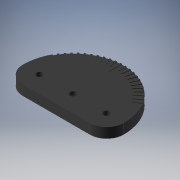
# Autodesk Inventor part: Angled Sensor Mount Base
Saved by Autodesk Inventor 2019 (Build 230136000, 136)
## iProperties
Created: 2019-01-21
Part Number: Angled Sensor Mount Base
Material: Generic
Document SubType Name: Modeling
Designer: Billy
Density: 1 g/cm^3
Appearance: Default
Author: Billy
Autodesk Inventor part; units mm, degrees
ref_plane "YZ Plane" through (0, 0, 0) normal (1, 0, 0) x (0, 1, 0)
ref_plane "XZ Plane" through (0, 0, 0) normal (0, 1, 0) x (-1, 0, 0)
ref_plane "XY Plane" through (0, 0, 0) normal (0, 0, 1) x (1, 0, 0)
sketch "Sketch1" plane through (0, 0, 0) normal (0, 1, 0) x (-1, 0, 0)
  circle A0 centre (0, 0) radius 2
  arc A1 (0, 10) -> (0, -10) centre (0, 0) ccw
  circle A2 centre (40, 0) radius 2
  arc A3 (40, -10) -> (40, 10) centre (40, 0) ccw
  line L0 (40, 10) -> (0, 10)
  line L1 (40, -10) -> (0, -10)
  circle A4 centre (20, 0) radius 2
  dimension "d0" = 4
  dimension "d1" = 20
  dimension "d2" = 4
  dimension "d3" = 20
  dimension "d4" = 4
  constraints: 5 centre point, 4 end point, 4 point on circle, 3 coincident, 1 parallel, 1 tangent
  measures "d0" diameter of A0
  measures "d1" diameter of A1
  measures "d2" diameter of A2
  measures "d3" diameter of A3
  measures "d4" diameter of A4
extrude "Extrusion1" add sketch "Sketch1" along normal blind 6
sketch "Sketch2" plane through (0, 0, 0) normal (0, -1, 0) x (1, 0, 0)
  circle A0 centre (-20, 0) radius 2 projected
  circle A1 centre (-40, 0) radius 2 projected
  circle A2 centre (0, 0) radius 2 projected
  arc A3 (-40, 10) -> (-40, -10) centre (-40, 0) ccw projected
  line L0 (-40, -10) -> (0, -10) projected
  arc A4 (0, -10) -> (0, 10) centre (0, 0) ccw projected
  line L1 (0, 10) -> (-40, 10) projected
  circle A5 centre (-20, 0) radius 5
  dimension "d7" = 10
  constraints: 1 centre point, 1 coincident
  measures "d7" diameter of A5
extrude "Extrusion2" cut sketch "Sketch2" against normal blind 4 contours A5
sketch "Sketch3" plane through (0, 6, 0) normal (0, 1, 0) x (1, 0, 0)
  circle A0 centre (-20, 0) radius 2
  circle A1 centre (-40, 0) radius 2
  circle A2 centre (0, 0) radius 2
  arc A3 (-40, 10) -> (-50, 0) centre (-40, 0) ccw
  line L0 (-40, -10) -> (0, -10)
  arc A4 (10, 0) -> (0, 10) centre (0, 0) ccw
  line L1 (0, 10) -> (-40, 10)
  arc A5 (10, 0) -> (-50, 0) centre (-20, 0) ccw
  constraints: 10 centre point, 6 point on circle, 4 end point, 1 coincident
extrude "Extrusion3" add sketch "Sketch3" against normal up to surface (6 mm away) contours A3 A5 A4 L1
sketch "Sketch4" plane through (0, 6, 0) normal (0, 1, 0) x (1, 0, 0)
  circle A0 centre (-20, 0) radius 2
  circle A1 centre (-40, 0) radius 2
  circle A2 centre (0, 0) radius 2
  arc A3 (-50, 0) -> (-40, -10) centre (-40, 0) ccw
  line L0 (-40, -10) -> (0, -10)
  arc A4 (0, -10) -> (10, 0) centre (0, 0) ccw
  arc A5 (-19, 29.9833) -> (-20, 30) centre (-20, 0) ccw
  arc A6 (-19, 29.9833) -> (-21, 29.9833) centre (-20, 0) ccw
  line L1 (-21, 29.9833) -> (-21, 25)
  line L2 (-21, 25) -> (-20, 25)
  line L3 (-19, 29.9833) -> (-19, 25)
  line L4 (-19, 25) -> (-20, 25)
  arc A7 (-21.8546, 29.9426) -> (-22.8517, 29.8642) centre (-20, 0) ccw
  arc A8 (-21.8546, 29.9426) -> (-23.8456, 29.7525) centre (-20, 0) ccw
  line L5 (-23.8456, 29.7525) -> (-23.3719, 24.7917)
  line L6 (-23.3719, 24.7917) -> (-22.3764, 24.8868)
  line L7 (-21.8546, 29.9426) -> (-21.3809, 24.9819)
  line L8 (-21.3809, 24.9819) -> (-22.3764, 24.8868)
  arc A9 (-24.6925, 29.6307) -> (-25.6775, 29.4579) centre (-20, 0) ccw
  arc A10 (-24.6925, 29.6307) -> (-26.6563, 29.2522) centre (-20, 0) ccw
  line L9 (-26.6563, 29.2522) -> (-25.7132, 24.359)
  line L10 (-25.7132, 24.359) -> (-24.7313, 24.5482)
  line L11 (-24.6925, 29.6307) -> (-23.7494, 24.7375)
  line L12 (-23.7494, 24.7375) -> (-24.7313, 24.5482)
  arc A11 (-27.4878, 29.0505) -> (-28.452, 28.7848) centre (-20, 0) ccw
  arc A12 (-27.4878, 29.0505) -> (-29.4068, 28.4871) centre (-20, 0) ccw
  line L13 (-29.4068, 28.4871) -> (-28.0028, 23.7056)
  line L14 (-28.0028, 23.7056) -> (-27.0433, 23.9873)
  line L15 (-27.4878, 29.0505) -> (-26.0838, 24.2691)
  line L16 (-26.0838, 24.2691) -> (-27.0433, 23.9873)
  arc A13 (-30.2153, 28.2072) -> (-31.1499, 27.851) centre (-20, 0) ccw
  arc A14 (-30.2153, 28.2072) -> (-32.072, 27.4639) centre (-20, 0) ccw
  line L17 (-32.072, 27.4639) -> (-30.2199, 22.8375)
  line L18 (-30.2199, 22.8375) -> (-29.2916, 23.2092)
  line L19 (-30.2153, 28.2072) -> (-28.3632, 23.5809)
  line L20 (-28.3632, 23.5809) -> (-29.2916, 23.2092)
  arc A15 (-32.8503, 27.1085) -> (-33.7468, 26.6651) centre (-20, 0) ccw
  arc A16 (-32.8503, 27.1085) -> (-34.628, 26.192) centre (-20, 0) ccw
  line L21 (-34.628, 26.192) -> (-32.3445, 21.7627)
  line L22 (-32.3445, 21.7627) -> (-31.4557, 22.2209)
  line L23 (-32.8503, 27.1085) -> (-30.5668, 22.6791)
  line L24 (-30.5668, 22.6791) -> (-31.4557, 22.2209)
  arc A17 (-35.369, 25.7642) -> (-36.2192, 25.2376) centre (-20, 0) ccw
  arc A18 (-35.369, 25.7642) -> (-37.0515, 24.6829) centre (-20, 0) ccw
  line L25 (-37.0515, 24.6829) -> (-34.3573, 20.4907)
  line L26 (-34.3573, 20.4907) -> (-33.516, 21.0313)
  line L27 (-35.369, 25.7642) -> (-32.6748, 21.572)
  line L28 (-32.6748, 21.572) -> (-33.516, 21.0313)
  arc A19 (-37.7484, 24.1866) -> (-38.5448, 23.5816) centre (-20, 0) ccw
  arc A20 (-37.7484, 24.1866) -> (-39.3205, 22.9503) centre (-20, 0) ccw
  line L29 (-39.3205, 22.9503) -> (-36.24, 19.0332)
  line L30 (-36.24, 19.0332) -> (-35.454, 19.6513)
  line L31 (-37.7484, 24.1866) -> (-34.6679, 20.2695)
  line L32 (-34.6679, 20.2695) -> (-35.454, 19.6513)
  arc A21 (-39.9671, 22.39) -> (-40.7024, 21.712) centre (-20, 0) ccw
  arc A22 (-39.9671, 22.39) -> (-41.4146, 21.0099) centre (-20, 0) ccw
  line L33 (-41.4146, 21.0099) -> (-37.9757, 17.4033)
  line L34 (-37.9757, 17.4033) -> (-37.252, 18.0934)
  line L35 (-39.9671, 22.39) -> (-36.5282, 18.7834)
  line L36 (-36.5282, 18.7834) -> (-37.252, 18.0934)
  arc A23 (-42.005, 20.3907) -> (-42.6725, 19.6458) centre (-20, 0) ccw
  arc A24 (-42.005, 20.3907) -> (-43.3147, 18.8792) centre (-20, 0) ccw
  line L37 (-43.3147, 18.8792) -> (-39.5486, 15.6158)
  line L38 (-39.5486, 15.6158) -> (-38.8937, 16.3715)
  line L39 (-42.005, 20.3907) -> (-38.2389, 17.1273)
  line L40 (-38.2389, 17.1273) -> (-38.8937, 16.3715)
  arc A25 (-43.8436, 18.2066) -> (-44.4373, 17.4017) centre (-20, 0) ccw
  arc A26 (-43.8436, 18.2066) -> (-45.0038, 16.5775) centre (-20, 0) ccw
  line L41 (-45.0038, 16.5775) -> (-40.9445, 13.6868)
  line L42 (-40.9445, 13.6868) -> (-40.3644, 14.5014)
  line L43 (-43.8436, 18.2066) -> (-39.7843, 15.316)
  line L44 (-39.7843, 15.316) -> (-40.3644, 14.5014)
  arc A27 (-45.4663, 15.8577) -> (-45.9808, 15) centre (-20, 0) ccw
  arc A28 (-45.4663, 15.8577) -> (-46.4663, 14.1256) centre (-20, 0) ccw
  line L45 (-46.4663, 14.1256) -> (-42.1506, 11.634)
  line L46 (-42.1506, 11.634) -> (-41.6506, 12.5)
  line L47 (-45.4663, 15.8577) -> (-41.1506, 13.366)
  line L48 (-41.1506, 13.366) -> (-41.6506, 12.5)
  arc A29 (-16.1544, 29.7525) -> (-17.1483, 29.8642) centre (-20, 0) ccw
  arc A30 (-16.1544, 29.7525) -> (-18.1454, 29.9426) centre (-20, 0) ccw
  line L49 (-18.1454, 29.9426) -> (-18.6191, 24.9819)
  line L50 (-18.6191, 24.9819) -> (-17.6236, 24.8868)
  line L51 (-16.6281, 24.7917) -> (-17.6236, 24.8868)
  line L52 (-16.1544, 29.7525) -> (-16.6281, 24.7917)
  arc A31 (-13.3437, 29.2522) -> (-14.3225, 29.4579) centre (-20, 0) ccw
  arc A32 (-13.3437, 29.2522) -> (-15.3075, 29.6307) centre (-20, 0) ccw
  line L53 (-15.3075, 29.6307) -> (-16.2506, 24.7375)
  line L54 (-16.2506, 24.7375) -> (-15.2687, 24.5482)
  line L55 (-14.2868, 24.359) -> (-15.2687, 24.5482)
  line L56 (-13.3437, 29.2522) -> (-14.2868, 24.359)
  arc A33 (-10.5932, 28.4871) -> (-11.548, 28.7848) centre (-20, 0) ccw
  arc A34 (-10.5932, 28.4871) -> (-12.5122, 29.0505) centre (-20, 0) ccw
  line L57 (-12.5122, 29.0505) -> (-13.9162, 24.2691)
  line L58 (-13.9162, 24.2691) -> (-12.9567, 23.9873)
  line L59 (-11.9972, 23.7056) -> (-12.9567, 23.9873)
  line L60 (-10.5932, 28.4871) -> (-11.9972, 23.7056)
  arc A35 (-7.928, 27.4639) -> (-8.8501, 27.851) centre (-20, 0) ccw
  arc A36 (-7.928, 27.4639) -> (-9.7847, 28.2072) centre (-20, 0) ccw
  line L61 (-9.7847, 28.2072) -> (-11.6368, 23.5809)
  line L62 (-11.6368, 23.5809) -> (-10.7084, 23.2092)
  line L63 (-9.7801, 22.8375) -> (-10.7084, 23.2092)
  line L64 (-7.928, 27.4639) -> (-9.7801, 22.8375)
  arc A37 (-5.372, 26.192) -> (-6.2532, 26.6651) centre (-20, 0) ccw
  arc A38 (-5.372, 26.192) -> (-7.1497, 27.1085) centre (-20, 0) ccw
  line L65 (-7.1497, 27.1085) -> (-9.4332, 22.6791)
  line L66 (-9.4332, 22.6791) -> (-8.5443, 22.2209)
  line L67 (-7.6555, 21.7627) -> (-8.5443, 22.2209)
  line L68 (-5.372, 26.192) -> (-7.6555, 21.7627)
  arc A39 (-2.9485, 24.6829) -> (-3.7808, 25.2376) centre (-20, 0) ccw
  arc A40 (-2.9485, 24.6829) -> (-4.631, 25.7642) centre (-20, 0) ccw
  line L69 (-4.631, 25.7642) -> (-7.3252, 21.572)
  line L70 (-7.3252, 21.572) -> (-6.484, 21.0313)
  line L71 (-5.6427, 20.4907) -> (-6.484, 21.0313)
  line L72 (-2.9485, 24.6829) -> (-5.6427, 20.4907)
  arc A41 (-0.6795, 22.9503) -> (-1.4552, 23.5816) centre (-20, 0) ccw
  arc A42 (-0.6795, 22.9503) -> (-2.2516, 24.1866) centre (-20, 0) ccw
  line L73 (-2.2516, 24.1866) -> (-5.3321, 20.2695)
  line L74 (-5.3321, 20.2695) -> (-4.546, 19.6513)
  line L75 (-3.76, 19.0332) -> (-4.546, 19.6513)
  line L76 (-0.6795, 22.9503) -> (-3.76, 19.0332)
  arc A43 (1.4146, 21.0099) -> (0.7024, 21.712) centre (-20, 0) ccw
  arc A44 (1.4146, 21.0099) -> (-0.0329, 22.39) centre (-20, 0) ccw
  line L77 (-0.0329, 22.39) -> (-3.4718, 18.7834)
  line L78 (-3.4718, 18.7834) -> (-2.748, 18.0934)
  line L79 (-2.0243, 17.4033) -> (-2.748, 18.0934)
  line L80 (1.4146, 21.0099) -> (-2.0243, 17.4033)
  arc A45 (3.3147, 18.8792) -> (2.6725, 19.6458) centre (-20, 0) ccw
  arc A46 (3.3147, 18.8792) -> (2.005, 20.3907) centre (-20, 0) ccw
  line L81 (2.005, 20.3907) -> (-1.7611, 17.1273)
  line L82 (-1.7611, 17.1273) -> (-1.1063, 16.3715)
  line L83 (-0.4514, 15.6158) -> (-1.1063, 16.3715)
  line L84 (3.3147, 18.8792) -> (-0.4514, 15.6158)
  arc A47 (5.0038, 16.5775) -> (4.4373, 17.4017) centre (-20, 0) ccw
  arc A48 (5.0038, 16.5775) -> (3.8436, 18.2066) centre (-20, 0) ccw
  line L85 (3.8436, 18.2066) -> (-0.2157, 15.316)
  line L86 (-0.2157, 15.316) -> (0.3644, 14.5014)
  line L87 (0.9445, 13.6868) -> (0.3644, 14.5014)
  line L88 (5.0038, 16.5775) -> (0.9445, 13.6868)
  arc A49 (6.4663, 14.1256) -> (5.9808, 15) centre (-20, 0) ccw
  arc A50 (6.4663, 14.1256) -> (5.4663, 15.8577) centre (-20, 0) ccw
  line L89 (5.4663, 15.8577) -> (1.1506, 13.366)
  line L90 (1.1506, 13.366) -> (1.6506, 12.5)
  line L91 (2.1506, 11.634) -> (1.6506, 12.5)
  line L92 (6.4663, 14.1256) -> (2.1506, 11.634)
  point P0 (-19, 25)
  point P1 (-16.6281, 24.7917)
  point P2 (-9.7801, 22.8375)
  point P3 (-7.6555, 21.7627)
  point P4 (-5.6427, 20.4907)
  point P5 (-3.76, 19.0332)
  point P6 (-2.0243, 17.4033)
  point P7 (0.9445, 13.6868)
  dimension "d17" = 60
  dimension "d21" = 60
  constraints: 186 end point, 119 point on circle, 78 centre point, 321 other
extrude "Extrusion4" cut sketch "Sketch4" against normal blind 0.5 contours L3 L4 L2 L1 A6 A5 | L7 L8 L6 L5 A8 A7 | L11 L12 L10 L9 A10 A9 | L15 L16 L14 L13 A12 A11 | L19 L20 L18 L17 A14 A13 | L23 L24 L22 L21 A16 A15 | L27 L28 L26 L25 A18 A17 | L31 L32 L30 L29 A20 A19 | L35 L36 L34 L33 A22 A21 | L39 L40 L38 L37 A24 A23 | L43 L44 L42 L41 A26 A25 | L47 L48 L46 L45 A28 A27 | L52 L51 L50 L49 A30 A29 | L56 L55 L54 L53 A32 A31 | L60 L59 L58 L57 A34 A33 | L64 L63 L62 L61 A36 A35 | L68 L67 L66 L65 A38 A37 | L72 L71 L70 L69 A40 A39 | L76 L75 L74 L73 A42 A41 | L80 L79 L78 L77 A44 A43 | L84 L83 L82 L81 A46 A45 | L88 L87 L86 L85 A48 A47 | L92 L91 L90 L89 A50 A49
sketch "Sketch5" plane through (0, 6, 0) normal (0, 1, 0) x (1, 0, 0)
  line L0 (-16.2506, 24.7375) -> (-15.3075, 29.6307) projected
  arc A0 (-15.3075, 29.6307) -> (-16.1544, 29.7525) centre (-20, 0) ccw projected
  line L1 (-16.1544, 29.7525) -> (-16.6281, 24.7917) projected
  line L2 (-16.6281, 24.7917) -> (-18.6191, 24.9819) projected
  line L3 (-18.6191, 24.9819) -> (-18.1454, 29.9426) projected
  arc A1 (-18.1454, 29.9426) -> (-19, 29.9833) centre (-20, 0) ccw projected
  line L4 (-19, 29.9833) -> (-19, 25) projected
  line L5 (-19, 25) -> (-21, 25) projected
  line L6 (-21, 25) -> (-21, 29.9833) projected
  arc A2 (-21, 29.9833) -> (-21.8546, 29.9426) centre (-20, 0) ccw projected
  line L7 (-21.8546, 29.9426) -> (-21.3809, 24.9819) projected
  line L8 (-21.3809, 24.9819) -> (-23.3719, 24.7917) projected
  line L9 (-23.3719, 24.7917) -> (-23.8456, 29.7525) projected
  arc A3 (-23.8456, 29.7525) -> (-24.6925, 29.6307) centre (-20, 0) ccw projected
  line L10 (-24.6925, 29.6307) -> (-23.7494, 24.7375) projected
  line L11 (-23.7494, 24.7375) -> (-25.7132, 24.359) projected
  line L12 (-25.7132, 24.359) -> (-26.6563, 29.2522) projected
  arc A4 (-26.6563, 29.2522) -> (-27.4878, 29.0505) centre (-20, 0) ccw projected
  line L13 (-27.4878, 29.0505) -> (-26.0838, 24.2691) projected
  line L14 (-26.0838, 24.2691) -> (-28.0028, 23.7056) projected
  line L15 (-28.0028, 23.7056) -> (-29.4068, 28.4871) projected
  arc A5 (-29.4068, 28.4871) -> (-30.2153, 28.2072) centre (-20, 0) ccw projected
  line L16 (-30.2153, 28.2072) -> (-28.3632, 23.5809) projected
  line L17 (-28.3632, 23.5809) -> (-30.2199, 22.8375) projected
  line L18 (-30.2199, 22.8375) -> (-32.072, 27.4639) projected
  arc A6 (-32.072, 27.4639) -> (-32.8503, 27.1085) centre (-20, 0) ccw projected
  line L19 (-32.8503, 27.1085) -> (-30.5668, 22.6791) projected
  line L20 (-30.5668, 22.6791) -> (-32.3445, 21.7627) projected
  line L21 (-32.3445, 21.7627) -> (-34.628, 26.192) projected
  arc A7 (-34.628, 26.192) -> (-35.369, 25.7642) centre (-20, 0) ccw projected
  line L22 (-35.369, 25.7642) -> (-32.6748, 21.572) projected
  line L23 (-32.6748, 21.572) -> (-34.3573, 20.4907) projected
  line L24 (-34.3573, 20.4907) -> (-37.0515, 24.6829) projected
  arc A8 (-37.0515, 24.6829) -> (-37.7484, 24.1866) centre (-20, 0) ccw projected
  line L25 (-37.7484, 24.1866) -> (-34.6679, 20.2695) projected
  line L26 (-34.6679, 20.2695) -> (-36.24, 19.0332) projected
  line L27 (-36.24, 19.0332) -> (-39.3205, 22.9503) projected
  arc A9 (-39.3205, 22.9503) -> (-39.9671, 22.39) centre (-20, 0) ccw projected
  line L28 (-39.9671, 22.39) -> (-36.5282, 18.7834) projected
  line L29 (-36.5282, 18.7834) -> (-37.9757, 17.4033) projected
  line L30 (-37.9757, 17.4033) -> (-41.4146, 21.0099) projected
  arc A10 (-41.4146, 21.0099) -> (-42.005, 20.3907) centre (-20, 0) ccw projected
  line L31 (-42.005, 20.3907) -> (-38.2389, 17.1273) projected
  line L32 (-38.2389, 17.1273) -> (-39.5486, 15.6158) projected
  line L33 (-39.5486, 15.6158) -> (-43.3147, 18.8792) projected
  arc A11 (-43.3147, 18.8792) -> (-43.8436, 18.2066) centre (-20, 0) ccw projected
  line L34 (-43.8436, 18.2066) -> (-39.7843, 15.316) projected
  line L35 (-39.7843, 15.316) -> (-40.9445, 13.6868) projected
  line L36 (-40.9445, 13.6868) -> (-45.0038, 16.5775) projected
  arc A12 (-45.0038, 16.5775) -> (-45.4663, 15.8577) centre (-20, 0) ccw projected
  line L37 (-45.4663, 15.8577) -> (-41.1506, 13.366) projected
  line L38 (-41.1506, 13.366) -> (-42.1506, 11.634) projected
  line L39 (-42.1506, 11.634) -> (-46.4663, 14.1256) projected
  arc A13 (-46.4663, 14.1256) -> (-50, 0) centre (-20, 0) ccw projected
  arc A14 (-50, 0) -> (-40, -10) centre (-40, 0) ccw projected
  line L40 (-40, -10) -> (0, -10) projected
  arc A15 (0, -10) -> (10, 0) centre (0, 0) ccw projected
  arc A16 (10, 0) -> (6.4663, 14.1256) centre (-20, 0) ccw projected
  line L41 (6.4663, 14.1256) -> (2.1506, 11.634) projected
  line L42 (2.1506, 11.634) -> (1.1506, 13.366) projected
  line L43 (1.1506, 13.366) -> (5.4663, 15.8577) projected
  arc A17 (5.4663, 15.8577) -> (5.0038, 16.5775) centre (-20, 0) ccw projected
  line L44 (5.0038, 16.5775) -> (0.9445, 13.6868) projected
  line L45 (0.9445, 13.6868) -> (-0.2157, 15.316) projected
  line L46 (-0.2157, 15.316) -> (3.8436, 18.2066) projected
  arc A18 (3.8436, 18.2066) -> (3.3147, 18.8792) centre (-20, 0) ccw projected
  line L47 (3.3147, 18.8792) -> (-0.4514, 15.6158) projected
  line L48 (-0.4514, 15.6158) -> (-1.7611, 17.1273) projected
  line L49 (-1.7611, 17.1273) -> (2.005, 20.3907) projected
  arc A19 (2.005, 20.3907) -> (1.4146, 21.0099) centre (-20, 0) ccw projected
  line L50 (1.4146, 21.0099) -> (-2.0243, 17.4033) projected
  line L51 (-2.0243, 17.4033) -> (-3.4718, 18.7834) projected
  line L52 (-3.4718, 18.7834) -> (-0.0329, 22.39) projected
  arc A20 (-0.0329, 22.39) -> (-0.6795, 22.9503) centre (-20, 0) ccw projected
  line L53 (-0.6795, 22.9503) -> (-3.76, 19.0332) projected
  line L54 (-3.76, 19.0332) -> (-5.3321, 20.2695) projected
  line L55 (-5.3321, 20.2695) -> (-2.2516, 24.1866) projected
  arc A21 (-2.2516, 24.1866) -> (-2.9485, 24.6829) centre (-20, 0) ccw projected
  line L56 (-2.9485, 24.6829) -> (-5.6427, 20.4907) projected
  line L57 (-5.6427, 20.4907) -> (-7.3252, 21.572) projected
  line L58 (-7.3252, 21.572) -> (-4.631, 25.7642) projected
  arc A22 (-4.631, 25.7642) -> (-5.372, 26.192) centre (-20, 0) ccw projected
  line L59 (-5.372, 26.192) -> (-7.6555, 21.7627) projected
  line L60 (-7.6555, 21.7627) -> (-9.4332, 22.6791) projected
  line L61 (-9.4332, 22.6791) -> (-7.1497, 27.1085) projected
  arc A23 (-7.1497, 27.1085) -> (-7.928, 27.4639) centre (-20, 0) ccw projected
  line L62 (-7.928, 27.4639) -> (-9.7801, 22.8375) projected
  line L63 (-9.7801, 22.8375) -> (-11.6368, 23.5809) projected
  line L64 (-11.6368, 23.5809) -> (-9.7847, 28.2072) projected
  arc A24 (-9.7847, 28.2072) -> (-10.5932, 28.4871) centre (-20, 0) ccw projected
  line L65 (-10.5932, 28.4871) -> (-11.9972, 23.7056) projected
  line L66 (-11.9972, 23.7056) -> (-13.9162, 24.2691) projected
  line L67 (-13.9162, 24.2691) -> (-12.5122, 29.0505) projected
  arc A25 (-12.5122, 29.0505) -> (-13.3437, 29.2522) centre (-20, 0) ccw projected
  line L68 (-13.3437, 29.2522) -> (-14.2868, 24.359) projected
  line L69 (-14.2868, 24.359) -> (-16.2506, 24.7375) projected
  circle A26 centre (-20, 0) radius 2 projected
  circle A27 centre (-40, 0) radius 2 projected
  circle A28 centre (0, 0) radius 2 projected
  line L70 (-21, 25) -> (-19, 25)
  line L71 (-19, 25) -> (-19, 22)
  line L72 (-19, 22) -> (-21, 22)
  line L73 (-21, 22) -> (-21, 25)
  dimension "d25" = 3
  constraints: 8 end point, 2 parallel, 1 horizontal, 1 perpendicular
  measures "d25" distance of L70.end L71.end
extrude "Extrusion5" cut sketch "Sketch5" against normal blind 0.5 contours L71 L72 L73 L5
body "Solid1"
